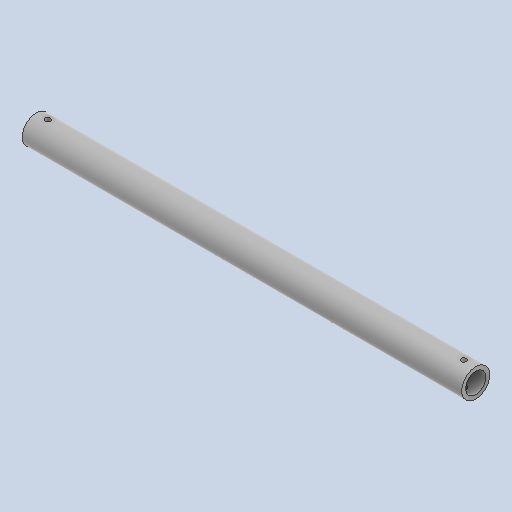
# Autodesk Inventor part: roller-hand-v1-roller
Saved by Autodesk Inventor 2025.1 (Build 291241000, 241)
## iProperties
Created: 2024-10-01
Part Number: roller-hand-v1-roller
Material: PVC 配管
Document SubType Name: Modeling
Designer: haruy
Density: 1.4 g/cm^3
Appearance: 滑らか - 標準の灰色
Author: haruy
Autodesk Inventor part; units mm, degrees
ref_plane "YZ Plane" through (0, 0, 0) normal (1, 0, 0) x (0, 1, 0)
ref_plane "XY Plane" through (0, 0, 0) normal (0, 0, 1) x (1, 0, 0)
sketch "スケッチ1" plane through (0, 0, 0) normal (1, 0, 0) x (0, 1, 0)
  circle A0 centre (0, 0) radius 9
  circle A1 centre (0, 0) radius 6.5
  dimension "d0" = 18
  dimension "d1" = 13
  constraints: 2 centre point, 2 coincident
  measures "d0" diameter of A0
  measures "d1" diameter of A1
extrude "押し出し1" add sketch "スケッチ1" along normal blind 280
ref_plane "作業平面1" through (0, -9, 0) normal (0, 1, 0) x (-1, 0, 0)
sketch "スケッチ2" plane through (0, -9, 0) normal (0, 1, 0) x (-1, 0, 0)
  line L0 (0, 9) -> (0, -9) projected
  line L1 (-280, 9) -> (-280, -9) projected
  point P0 (0, 0)
  point P1 (-7.5, 0)
  point P2 (-272.5, 0)
  dimension "d4" = 7.5
  dimension "d5" = 7.5
  measures "d4" distance from line of point (-7.5, 0) L0
  measures "d5" distance from line of L1 point (-272.5, 0)
hole "穴1" at (7.5, -9, 0) at (272.5, -9, 0) direction (0, 1, 0) diameter 3.4 end through all
